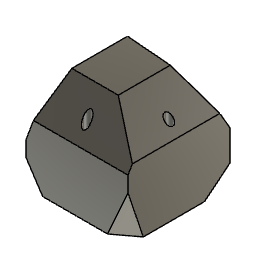
Suètone-drawing-object-02 v25 (Autodesk Fusion 360 design; units mm, degrees)
Autodesk Fusion 360 part; units mm, degrees
sketch "Esquisse1" plane through (0, 0, 0) normal (0, 0, 1) x (1, 0, 0)
  line L0 (50, 50) -> (-50, 50)
  line L1 (-50, 50) -> (-50, -50)
  line L2 (-50, -50) -> (50, -50)
  line L3 (50, -50) -> (50, 50)
  line L4 (50, 50) -> (-50, -50) construction
  line L5 (-50, 50) -> (50, -50) construction
  dimension "d1" = 100
  dimension "d2" = 100
  constraint horizontal L0
  constraint perpendicular L0 L1
  constraint parallel L0 L2
  constraint parallel L1 L3
  constraint coincident L4 origin
  constraint coincident L5 origin
  measures "d1" distance of L1.end L2.end
  measures "d2" distance of L0.end L1.end
extrude "Extrusion1" add sketch "Esquisse1" along normal blind 100 makes body 1
sketch "Esquisse2" plane through (50, 0, 0) normal (1, 0, 0) x (0, 1, 0)
  line L0 (-50, 0) -> (50, 0)
  line L1 (50, 0) -> (50, 100)
  line L2 (50, 100) -> (-50, 100)
  line L3 (-50, 100) -> (-50, 0)
  line L4 (-50, 67.3848) -> (50, 67.3848)
  constraint coincident L3 L4.start
  constraint coincident L1 L4.end
  constraint perpendicular L1 L4
ref_plane "Plan de construction1" through (50, 0, 67.3848) normal (0.707107, 0, 0.707107) x (0, 1, 0)
split "Scinder1" by plane through (50, 0, 67.3848) normal (0.707107, 0, 0.707107) bodies 1 makes body 2 at (39.1283, -16.6667, 100)
sketch "Esquisse3" plane through (0, 50, 0) normal (0, 1, 0) x (-1, 0, 0)
  line L0 (-17.3848, 100) -> (-50, 67.3848)
  line L1 (-50, 67.3848) -> (-50, 0)
  line L2 (-50, 0) -> (50, 0)
  line L3 (50, 0) -> (50, 100)
  line L4 (50, 100) -> (-17.3848, 100)
  line L5 (-50, 50) -> (50, 64.0079)
  constraint coincident L1 L5.start
  constraint coincident L3 L5.end
ref_plane "Plan de construction2" through (0, 50, 57.0039) normal (0.069362, 0.866025, 0.495166) x (-0.990331, 0, 0.138724)
split "Scinder2" by plane through (0, 50, 57.0039) normal (0.069362, 0.866025, 0.495166) bodies 1 makes body 3 at (5.7949, 50, 71.336)
sketch "Esquisse4" plane through (0, -50, 0) normal (0, -1, 0) x (1, 0, 0)
  line L0 (50, 67.3848) -> (17.3848, 100)
  line L1 (17.3848, 100) -> (-50, 100)
  line L2 (-50, 100) -> (-50, 0)
  line L3 (-50, 0) -> (50, 0)
  line L4 (50, 0) -> (50, 67.3848)
  line L5 (50, 60) -> (-50, 60)
  constraint coincident L4 L5.start
  constraint coincident L2 L5.end
  constraint perpendicular L2 L5
ref_plane "Plan de construction3" through (0, -50, 60) normal (0, -0.866025, 0.5) x (-1, 0, 0)
split "Scinder3" by plane through (0, -50, 60) normal (0, -0.866025, 0.5) bodies 1 makes body 4 at (5.7949, -50, 73.3333)
delete_body "RemoveBody1" bodies 2
delete_body "RemoveBody2" bodies 3
delete_body "RemoveBody3" bodies 4
sketch "Esquisse5" plane through (-50, 0, 0) normal (-1, 0, 0) x (0, -1, 0)
  line L0 (50, 60) -> (26.906, 100)
  line L1 (26.906, 100) -> (-29.4208, 100)
  line L2 (-29.4208, 100) -> (-50, 64.0079)
  line L3 (-50, 64.0079) -> (-50, 0)
  line L4 (-50, 0) -> (50, 0)
  line L5 (50, 0) -> (50, 60)
  line L6 (50, 40) -> (-50, 40)
  constraint coincident L5 L6.start
  constraint coincident L3 L6.end
  constraint perpendicular L3 L6
ref_plane "Plan de construction4" through (-50, 0, 40) normal (-0.939693, 0, 0.34202) x (0, 1, 0)
split "Scinder4" by plane through (-50, 0, 40) normal (-0.939693, 0, 0.34202) bodies 1 makes body 5 at (-50, -8.9687, 74.6693)
delete_body "RemoveBody4" bodies 5
sketch "Esquisse6" plane through (0, 50, 0) normal (0, 1, 0) x (-1, 0, 0)
  line L0 (50, 40) -> (41.6858, 62.8432)
  line L1 (41.6858, 62.8432) -> (-50, 50)
  line L2 (-50, 50) -> (-50, 0)
  line L3 (-50, 0) -> (50, 0)
  line L4 (50, 0) -> (50, 40)
  line L5 (-50, 15) -> (50, 15)
  line L6 (50, 0, -100) -> (50, 40, -100)
  line L7 (50, 15, -100) -> (50, 15, 0)
  line L8 (-50, 0, -100) -> (-50, 60, -100)
  line L9 (50, 15, -100) -> (-50, 15, -100)
  line L10 (-50, 15, -100) -> (-50, 15, 0)
  constraint coincident L2 L5.start
  constraint coincident L4 L5.end
  constraint perpendicular L4 L5
sketch "Esquisse7" plane through (0, -63.4808, 36.6506) normal (0, -0.866025, 0.5) x (1, 0, 0)
  line L0 (-28.1618, 73.1495) -> (-42.7206, 26.9615)
  line L1 (-42.7206, 26.9615) -> (50, 26.9615)
  line L2 (50, 26.9615) -> (50, 35.4887)
  line L3 (50, 35.4887) -> (17.3848, 73.1495)
  line L4 (17.3848, 73.1495) -> (-28.1618, 73.1495)
  line L5 (33.6924, 54.3191) -> (22.5947, 26.9615)
  constraint midpoint L3 L5.start
  constraint coincident L1 L5.end
ref_plane "Plan de construction9" through (28.1435, -43.1606, 71.8462) normal (0.46333, -0.843975, 0.270242) x (-0.375902, -0.46333, -0.802511)
sketch "Esquisse8" plane through (4.9613, 61.9448, 35.418) normal (0.069362, 0.866025, 0.495166) x (-0.996808, 0.079837, 0)
  line L0 (45.5445, 31.5668) -> (30.2811, 74.3348)
  line L1 (30.2811, 74.3348) -> (-15.4113, 74.3348)
  line L2 (-15.4113, 74.3348) -> (-46.6421, 36.7942)
  line L3 (-46.6421, 36.7942) -> (-45.8486, 16.7841)
  line L4 (-45.8486, 16.7841) -> (45.5445, 31.5668)
  line L5 (-46.6421, 36.7942) -> (-22.3107, 19.7571)
  line L6 (-46.6421, 36.7942) -> (-16.9389, 36.7942) construction
  dimension "d14" = 35
  constraint horizontal L6
  constraint coincident L2.end L3.start
  measures "d14" angle of L5 L6
ref_plane "Plan de construction10" through (38.2098, 45.2358, 59.9839) normal (0.295172, 0.937306, 0.185285) x (-0.793862, 0.348507, -0.498322)
sketch "Esquisse9" plane through (-57.0069, 0, 20.7488) normal (-0.939693, 0, 0.34202) x (0, -1, 0)
  line L0 (-50, 20.4867) -> (50, 20.4867)
  line L1 (50, 20.4867) -> (50, 41.7703)
  line L2 (50, 41.7703) -> (26.906, 84.3374)
  line L3 (26.906, 84.3374) -> (-27.6718, 84.3374)
  line L4 (-27.6718, 84.3374) -> (-50, 44.7959)
  line L5 (-50, 44.7959) -> (-50, 20.4867)
ref_plane "Plan de construction11" through (-50, 0, 40) normal (-0.766044, 0, 0.642788) x (0, -1, 0)
sketch "Esquisse13" plane through (0, 0, 0) normal (0, 0, 1) x (1, 0, 0)
  circle A0 centre (0, 40) radius 4
  circle A1 centre (-40, 0) radius 4
  circle A2 centre (0, -40) radius 4
  circle A3 centre (40, 0) radius 4
  dimension "d24" = 8
  dimension "d26" = 360
  measures "d24" diameter of A0
extrude "Extrusion4" cut sketch "Esquisse13" along normal blind 110 bodies 1
sketch "Esquisse14" plane through (-50, 0, 0) normal (-1, 0, 0) x (0, -1, 0)
  line L0 (50, 40) -> (-50, 40)
  line L1 (-50, 40) -> (-50, 0)
  line L2 (-50, 0) -> (50, 0)
  line L3 (50, 0) -> (50, 40)
  line L4 (50, 25) -> (28.3706, 0)
  constraint coincident L3 L4.start
  constraint coincident L2 L4.end
ref_plane "Plan de construction12" through (-50, -39.1853, 12.5) normal (0.707107, 0.534747, 0.46265) x (0, 0.654286, -0.756247)
split "Scinder12" by plane through (-50, -39.1853, 12.5) normal (0.707107, 0.534747, 0.46265) bodies 1 makes body 6 at (-0.0996, 12.0037, 0)
delete_body "RemoveBody12" bodies 1
sketch "Esquisse15" plane through (0, 0, 0) normal (0, 0, -1) x (1, 0, 0)
  line L0 (-33.6428, 50) -> (-50, 28.3706)
  line L1 (-50, 28.3706) -> (-50, -50)
  line L2 (-50, -50) -> (50, -50)
  line L3 (50, -50) -> (50, 50)
  line L4 (50, 50) -> (-33.6428, 50)
  circle A0 centre (0, 40) radius 4
  circle A1 centre (40, 0) radius 4
  circle A2 centre (-40, 0) radius 4
  circle A3 centre (0, -40) radius 4
  line L5 (50, -25) -> (15, -50)
  constraint coincident L3 L5.start
  constraint coincident L2 L5.end
ref_plane "Plan de construction13" through (32.5, 37.5, 0) normal (-0.410997, -0.575396, 0.707107) x (-0.813733, 0.581238, 0)
split "Scinder13" by plane through (32.5, 37.5, 0) normal (-0.410997, -0.575396, 0.707107) bodies 6 makes body 7 at (-0.0996, 12.0037, 0)
delete_body "RemoveBody13" bodies 6
sketch "Esquisse16" plane through (0, 0, 0) normal (0, 0, -1) x (1, 0, 0)
  circle A0 centre (0, -40) radius 4
  circle A1 centre (-40, 0) radius 4
  circle A2 centre (40, 0) radius 4
  circle A3 centre (0, 40) radius 4
  line L0 (15, -50) -> (50, -25)
  line L1 (50, -25) -> (50, 50)
  line L2 (50, 50) -> (-33.6428, 50)
  line L3 (-33.6428, 50) -> (-50, 28.3706)
  line L4 (-50, 28.3706) -> (-50, -50)
  line L5 (-50, -50) -> (15, -50)
  line L6 (30, 50) -> (50, 35)
  constraint coincident L2 L6.start
  constraint coincident L1 L6.end
ref_plane "Plan de construction14" through (40, -42.5, 0) normal (-0.579555, 0.772741, 0.258819) x (0.8, 0.6, 0)
split "Scinder14" by plane through (40, -42.5, 0) normal (-0.579555, 0.772741, 0.258819) bodies 7 makes body 8 at (-0.0996, 12.0037, 0)
delete_body "RemoveBody14" bodies 7
sketch "Esquisse17" plane through (0, 0, 0) normal (0, 0, -1) x (1, 0, 0)
  line L0 (50, 35) -> (30, 50)
  line L1 (30, 50) -> (-33.6428, 50)
  line L2 (-33.6428, 50) -> (-50, 28.3706)
  line L3 (-50, 28.3706) -> (-50, -50)
  line L4 (-50, -50) -> (15, -50)
  line L5 (15, -50) -> (50, -25)
  line L6 (50, -25) -> (50, 35)
  circle A0 centre (0, -40) radius 4
  circle A1 centre (-40, 0) radius 4
  circle A2 centre (40, 0) radius 4
  circle A3 centre (0, 40) radius 4
  line L7 (-31.6831, -50) -> (-50, -33.737)
  constraint coincident L4 L7.start
  constraint coincident L3 L7.end
ref_plane "Plan de construction15" through (-40.8416, 41.8685, 0) normal (0.641316, -0.722307, 0.258819) x (-0.747787, -0.663939, 0)
split "Scinder15" by plane through (-40.8416, 41.8685, 0) normal (0.641316, -0.722307, 0.258819) bodies 8 makes body 9 at (-0.0996, 12.0037, 0)
delete_body "RemoveBody15" bodies 8
